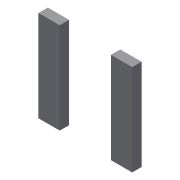
# Autodesk Inventor part: Fan_outlet_2
Saved by Autodesk Inventor 2017 (Build 210142000, 142)
## iProperties
Created: 2018-04-20
Part Number: Fan_outlet_2
Material: Generic
Document SubType Name: Modeling
Designer: Kathryn Rosie
Density: 1 g/cm^3
Appearance: Default
Author: Kathryn Rosie
Autodesk Inventor part; units mm, degrees
ref_plane "YZ Plane" through (0, 0, 0) normal (1, 0, 0) x (0, 1, 0)
ref_plane "XZ Plane" through (0, 0, 0) normal (0, 1, 0) x (-1, 0, 0)
ref_plane "XY Plane" through (0, 0, 0) normal (0, 0, 1) x (1, 0, 0)
sketch "Sketch1" plane through (0, 0, 0) normal (0, 0, 1) x (1, 0, 0)
  line L0 (-522, -25) -> (522, -25) projected
  circle A0 centre (210, 82) radius 55 projected
  line L1 (522, 189) -> (-522, 189) projected
  line L2 (100, -25) -> (150, -25)
  line L3 (150, -25) -> (150, 189)
  line L4 (150, 189) -> (100, 189)
  line L5 (100, 189) -> (100, -25)
  line L6 (210, 82) -> (210, -25) construction
  line L7 (320, -25) -> (270, -25)
  line L8 (270, -25) -> (270, 189)
  line L9 (270, 189) -> (320, 189)
  line L10 (320, 189) -> (320, -25)
  point P0 (0, 0)
  dimension "d0" = 50
  dimension "d1" = 60
  constraints: 18 end point, 4 symmetric about line, 3 point on line, 2 parallel, 2 perpendicular, 1 horizontal
  measures "d0" distance between parallel lines of L5 L3
  measures "d1" distance from line of L6.start L3
extrude "Extrusion1" add sketch "Sketch1" along normal blind 22 contours L5 L1 L3 L0 | L8 L1 L10 L0
body "Solid1"
